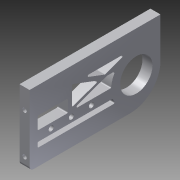
# Autodesk Inventor part: support_caterpillar_lateral_v3_Right
Saved by Autodesk Inventor 2015 (Build 190159000, 159)
## iProperties
Created: 2016-03-21
Part Number: support_caterpillar_lateral_v3_Right
Material: Plástico ABS
Document SubType Name: Modeling
Designer: JavierPC
Density: 1.06 g/cm^3
Appearance: Suave - Blanco
Author: JavierPC
Autodesk Inventor part; units mm, degrees
ref_plane "YZ Plane" through (0, 0, 0) normal (1, 0, 0) x (0, 1, 0)
ref_plane "XZ Plane" through (0, 0, 0) normal (0, 1, 0) x (-1, 0, 0)
ref_plane "XY Plane" through (0, 0, 0) normal (0, 0, 1) x (1, 0, 0)
sketch "Boceto1" plane through (0, 0, 0) normal (0, 1, 0) x (-1, 0, 0)
  line L0 (-2.5, 20) -> (2.5, 20)
  line L1 (2.5, 20) -> (2.5, -15)
  line L2 (2.5, -15) -> (-2.5, -15)
  line L3 (-2.5, -15) -> (-2.5, 20)
  line L4 (0, 20) -> (0, -15)
  line L5 (-2.5, 2.5) -> (2.5, 2.5)
  point P0 (0, 0)
  point P1 (0, 2.5)
  dimension "d0" = 5
  dimension "d1" = 35
  dimension "d26" = 20
  constraints: 12 end point, 5 midpoint, 2 parallel, 1 horizontal, 1 perpendicular, 1 vertical
  measures "d0" distance of L1.end L2.end
  measures "d1" distance of L0.end L1.end
  measures "d26" distance from line of point (0, 0) L0
extrude "Main Body" add sketch "Boceto1" along normal mid plane 100
sketch "Axles" plane through (0, 0, 0) normal (1, 0, 0) x (0, 1, 0)
  line L0 (50, 20) -> (-50, 20) projected
  circle A0 centre (38, 0) radius 8.05
  circle A1 centre (-40, 0) radius 6.5
  point P0 (0, 0)
  dimension "d53" = 5
  dimension "d55" = 13
  dimension "d11" = 20
  dimension "d12" = 40
  dimension "d13" = 38
  dimension "d14" = 20
  dimension "d22" = 16.1
  dimension "d23" = 13
  constraints: 2 centre point, 2 coincident
  measures "d11" distance from line of L0 point (-40, 0)
  measures "d12" distance of point (0, 0) point (-40, 0)
  measures "d13" distance of point (38, 0) point (0, 0)
  measures "d14" distance from line of L0 point (38, 0)
  measures "d22" diameter of A0
  measures "d23" diameter of A1
extrude "Bearings" cut sketch "Axles" along normal mid plane 100
sketch "Boceto4" plane through (0, 0, 0) normal (1, 0, 0) x (0, 1, 0)
  line L0 (-50.2028, -2.5) -> (5.4434, -2.5)
  line L1 (-50, -15) -> (-50, 20) projected
  line L2 (-50, 7.0921) -> (-15, 7.0921)
  line L3 (-15, 7.0921) -> (-15, -12.9079)
  line L4 (-15, -12.9079) -> (-50, -12.9079)
  line L5 (-50, -12.9079) -> (-50, 7.0921)
  point P0 (0, 0)
  dimension "d27" = 20
  dimension "d28" = 35
  constraints: 10 end point, 2 horizontal, 2 parallel, 1 perpendicular, 1 point on line
  measures "d27" distance between parallel lines of L4 L2
  measures "d28" distance of L2.start L2.end
sketch "Boceto5" plane through (0, 0, 0) normal (1, 0, 0) x (0, 1, 0)
  line L0 (-50, 25.8088) -> (-15, 25.8088)
  line L1 (-15, 25.8088) -> (-15, -24.1912)
  line L2 (-15, -24.1912) -> (-50, -24.1912)
  line L3 (-50, -24.1912) -> (-50, 25.8088)
  point P0 (0, 0)
  point P1 (-50, 20)
  dimension "d29" = 35
  dimension "d56" = 50
  constraints: 8 end point, 2 parallel, 1 horizontal, 1 perpendicular
  measures "d29" distance of L0.start L0.end
  measures "d56" distance of L2.end L0.start
extrude "Spring_support_space" cut sketch "Boceto5" along normal mid plane 10
sketch "Boceto6" plane through (-2.5, -15, 20) normal (0, -1, 0) x (1, 0, 0)
  line L0 (2.5, -16) -> (2.5, -24)
  line L1 (-2.5, -6.5) -> (-2.5, 6.5)
  line L2 (2.5, -20) -> (23.3777, -20)
  line L3 (2.5, 18.3522) -> (2.5, -26.5488)
  circle A0 centre (2.5, -10) radius 1.05
  circle A1 centre (2.5, -30) radius 1.05
  line L4 (0, 0) -> (5, 0) projected
  line L5 (0, 0) -> (5, 0) projected
  line L6 (0, -28.05) -> (0, -11.95) projected
  line L7 (5, -11.95) -> (5, -28.05) projected
  line L8 (0, -28.05) -> (5, -28.05) projected
  line L9 (0, -11.95) -> (5, -11.95) projected
  point P0 (2.5, 0)
  point P1 (0, -20)
  dimension "d35" = 2.1
  dimension "d36" = 20
  constraints: 8 end point, 3 midpoint, 3 point on line, 2 centre point, 1 horizontal, 1 symmetric about line, 1 vertical, 1 other
  measures "d35" diameter of A0
  measures "d36" diameter of A0.centre L2
extrude "Holes" cut sketch "Boceto6" against normal blind 15 contours A0 L3 | L3 A0 | A1
sketch "Boceto10" plane through (-2.5, -15, 20) normal (0, -1, 0) x (1, 0, 0)
  circle A0 centre (2.5, -10) radius 1.05 projected
  circle A1 centre (2.5, -30) radius 1.05 projected
  circle A2 centre (2.5, -10) radius 3.5
  line L0 (-5.1427, -20) -> (9.8665, -20)
  circle A3 centre (2.5, -30) radius 3.5
  point P0 (2.5, -20)
  dimension "d59" = 7
  constraints: 2 centre point, 2 end point, 1 coincident, 1 horizontal, 1 symmetric about line, 1 other
  measures "d59" diameter of A2
fillet "Edges" radius 15 1 edges at (0, 50, -15)
fillet "Edges" radius 2 1 edges at (0, -15, -15)
sketch "Boceto7" plane through (0, 0, 0) normal (1, 0, 0) x (0, 1, 0)
  line L0 (-15, -15) -> (-15, 20) projected
  line L1 (-50, 20) -> (50, 20) projected
  circle A0 centre (-8.5, 17) radius 1.2
  point P0 (0, 0)
  point P1 (45, 20)
  point P2 (-15, 15.1502)
  dimension "d41" = 6.5
  dimension "d42" = 3
  dimension "d50" = 2.4
  constraints: 1 centre point, 1 coincident
  measures "d41" distance from line of L0 point (-8.5, 17)
  measures "d42" distance from line of point (-8.5, 17) L1
  measures "d50" diameter of A0
extrude "Extrusión6" [suppressed]
pattern_linear "Patrón rectangular1" [suppressed]
sketch "Boceto8" plane through (0, 0, 0) normal (1, 0, 0) x (0, 1, 0)
  circle A0 centre (-4.2763, -1.9) radius 1.25 projected
  circle A1 centre (5.7237, -1.9) radius 1.25 projected
  circle A2 centre (15.7237, -1.9) radius 1.25 projected
  point P0 (0, 0)
extrude "Extrusión7" cut sketch "Boceto8" against normal up to surface (5 mm away) from surface at 2.5
sketch "Boceto11" plane through (2.5, -15, 20) normal (1, 0, 0) x (0, 0, -1)
  circle A0 centre (21.9, 10.7237) radius 1.25 projected
  circle A1 centre (21.9, 20.7237) radius 1.25 projected
  circle A2 centre (21.9, 30.7237) radius 1.25 projected
  line L0 (11.05, 0) -> (8.95, 0) projected
  line L1 (11.05, 15) -> (8.95, 15) projected
  line L2 (31.05, 0) -> (28.95, 0) projected
  line L3 (31.05, 15) -> (28.95, 15) projected
  line L4 (31.05, 0) -> (28.95, 0) projected
  line L5 (0, 0) -> (33, 0) projected
  circle A3 centre (20, 53) radius 8.05 projected
  line L6 (0, 65) -> (0, 0) projected
  line L7 (24.4, 19) -> (26.9, 19)
  line L8 (19.4, 20.9385) -> (19.4, 41.0847)
  line L9 (18.3253, 20) -> (18.3311, 20.0149)
  line L10 (20.4689, 19.9851) -> (20.4635, 20)
  line L11 (19.4, 20.9385) -> (13.1, 38.3464)
  arc A4 (13.1, 42.5769) -> (19.4, 40.5144) centre (20, 53) ccw
  arc A5 (24.4, 41.3) -> (26.9, 42.5769) centre (20, 53) ccw
  line L12 (13.1, 38.3464) -> (13.1, 42.5769)
  line L13 (24.4, 19) -> (24.4, 41.3)
  line L14 (26.9, 19) -> (26.9, 42.5769)
  line L15 (24.4, 19) -> (26.9, 19)
  line L16 (13.1, 4) -> (13.1, 19)
  line L17 (13.1, 34.4694) -> (8, 21)
  line L18 (8, 26.6481) -> (12.0549, 37.3572)
  line L19 (17.9746, 21) -> (13.1, 34.4694)
  line L20 (12.0549, 37.3572) -> (8, 48.5615)
  line L21 (8, 26.6481) -> (8, 48.5615)
  line L22 (13.1, 4) -> (19.4, 4)
  line L23 (24.4, 4) -> (26.9, 4)
  line L24 (24.4, 4) -> (24.4, 19)
  line L25 (26.9, 4) -> (26.9, 19)
  line L26 (19.4, 4) -> (19.4, 19)
  line L27 (13.1, 19) -> (19.4, 19)
  line L28 (8, 21) -> (17.9746, 21)
  point P0 (20, 15)
  point P1 (27.1716, 0)
  constraints: 44 end point, 9 vertical, 4 point on circle, 2 centre point, 2 horizontal, 1 coincident, 1 parallel, 1 point on line, 2 other
extrude "Extrusión9" cut sketch "Boceto11" against normal blind 10 contours L13 A5 L14 L7 | L7 L25 L23 L24 | L11 L12 A4 L8 | L16 L27 L26 L22 | L19 L28 L17 | L21 L20 L18
extrude "Extrusión10" [suppressed]
fillet "Empalme2" radius 0.5 18 edges at (0, 6, 2.0254) (0, 19.4694, 6.9) (0, 6, 12) (0, 22.3572, 7.9451) (0, 33.5615, 12) (0, 11.6481, 12) (0, -11, 0.6) (0, 4, 6.9) (0, -11, -6.9) (0, -11, -4.4) (0, 27.5769, -6.9) (0, 26.3, -4.4) (0, 25.5144, 0.6) (0, 27.5769, 6.9) (0, 23.3464, 6.9) (0, 5.9385, 0.6) (0, -11, 6.9) (0, 4, 0.6)
sketch "Boceto13" plane through (-2.5, -15, 20) normal (-1, 0, 0) x (0, 0, 1)
  circle A0 centre (-3, 58.5) radius 1.2 projected
  circle A1 centre (-3, 45.5) radius 1.2 projected
  circle A2 centre (-3, 32.5) radius 1.2 projected
  circle A3 centre (-3, 19.5) radius 1.2 projected
  circle A4 centre (-3, 6.5) radius 1.2 projected
  circle A5 centre (-21.9, 10.7237) radius 1.25 projected
  circle A6 centre (-21.9, 20.7237) radius 1.25 projected
  circle A7 centre (-21.9, 30.7237) radius 1.25 projected
  point P0 (-20, 15)
hole "Agujero4" at (-2.5, -4.2763, -1.9) at (-2.5, 5.7237, -1.9) at (-2.5, 15.7237, -1.9) direction (1, 0, 0) diameter 2.4 end through all countersink diameter 4.6 countersink angle 90
